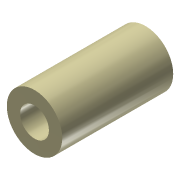
# Autodesk Inventor part: Nylon spacer 1 x 14-20
Saved by Autodesk Inventor 2013 (Build 170138000, 138)
## iProperties
Created: 2013-04-06
Part Number: Nylon spacer 1 x 14-20
Material: Nylon 6/6
Document SubType Name: Modeling
Designer: Niemitalo_Dan
Density: 1 g/cm^3
Author: Niemitalo_Dan
Autodesk Inventor part; units mm, degrees
ref_plane "YZ Plane" through (0, 0, 0) normal (1, 0, 0) x (0, 1, 0)
ref_plane "XZ Plane" through (0, 0, 0) normal (0, 1, 0) x (-1, 0, 0)
ref_plane "XY Plane" through (0, 0, 0) normal (0, 0, 1) x (1, 0, 0)
sketch "Sketch1" plane through (0, 0, 0) normal (0, 0, 1) x (1, 0, 0)
  circle A0 centre (0, 0) radius 3.302
  circle A1 centre (0, 0) radius 6.35
  dimension "d0" = 6.604
  dimension "d1" = 12.7
  constraints: 2 centre point, 2 coincident
  measures "d0" diameter of A0
  measures "d1" diameter of A1
extrude "Extrusion1" add sketch "Sketch1" along normal mid plane 25.4
body "Solid1"
